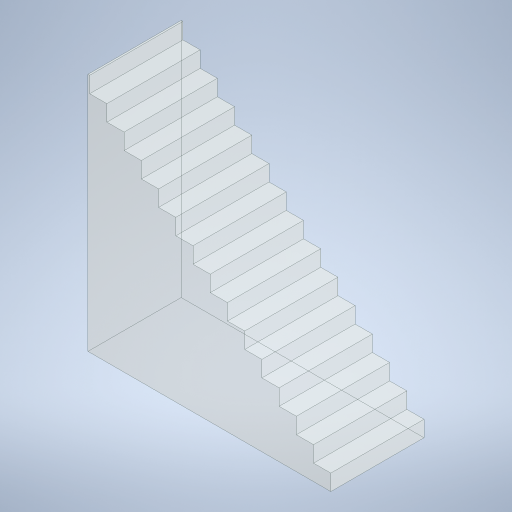
# Autodesk Inventor part: Stairs_Between_Finished_Basement_And_First_Floor
Saved by Autodesk Inventor 2024 (Build 280153000, 153)
## iProperties
Created: 2023-05-16
Part Number: Stairs_Between_Finished_Basement_And_First_Floor
Material: Steel
Document SubType Name: Modeling
Designer: Tom
Density: 7.85 g/cm^3
Appearance: Clear
Mass: 2.17052e+07 g
Surface Area: 147038 cm^2
Volume: 2.765e+06 cm^3
Author: Tom
Autodesk Inventor part; units mm, degrees
ref_plane "YZ Plane" through (0, 0, 0) normal (1, 0, 0) x (0, 1, 0)
ref_plane "XZ Plane" through (0, 0, 0) normal (0, 1, 0) x (-1, 0, 0)
ref_plane "XY Plane" through (0, 0, 0) normal (0, 0, 1) x (1, 0, 0)
sketch "Sketch1" plane through (0, 0, 0) normal (0, 0, 1) x (1, 0, 0)
  line L0 (-190.0464, 176.53) -> (-190.0464, 353.06)
  line L1 (-190.0464, 353.06) -> (-380.0929, 353.06)
  line L2 (-380.0929, 353.06) -> (-380.0929, 529.59)
  line L3 (-380.0929, 529.59) -> (-570.1393, 529.59)
  line L4 (-570.1393, 529.59) -> (-570.1393, 706.12)
  line L5 (-570.1393, 706.12) -> (-760.1857, 706.12)
  line L6 (-760.1857, 706.12) -> (-760.1857, 882.65)
  line L7 (-760.1857, 882.65) -> (-950.2321, 882.65)
  line L8 (-950.2321, 882.65) -> (-950.2321, 1059.18)
  line L9 (-950.2321, 1059.18) -> (-1140.2786, 1059.18)
  line L10 (-1140.2786, 1059.18) -> (-1140.2786, 1235.71)
  line L11 (-1140.2786, 1235.71) -> (-1330.325, 1235.71)
  line L12 (-1330.325, 1235.71) -> (-1330.325, 1412.24)
  line L13 (-1330.325, 1412.24) -> (-1520.3714, 1412.24)
  line L14 (-1520.3714, 1412.24) -> (-1520.3714, 1588.77)
  line L15 (-1520.3714, 1588.77) -> (-1710.4179, 1588.77)
  line L16 (-1710.4179, 1588.77) -> (-1710.4179, 1765.3)
  line L17 (-1710.4179, 1765.3) -> (-1900.4643, 1765.3)
  line L18 (-1900.4643, 1765.3) -> (-1900.4643, 1941.83)
  line L19 (-1900.4643, 1941.83) -> (-2090.5107, 1941.83)
  line L20 (-2090.5107, 1941.83) -> (-2090.5107, 2118.36)
  line L21 (-2090.5107, 2118.36) -> (-2280.5571, 2118.36)
  line L22 (-2280.5571, 2118.36) -> (-2280.5571, 2294.89)
  line L23 (-2280.5571, 2294.89) -> (-2470.6036, 2294.89)
  line L24 (-190.0464, 176.53) -> (0, 176.53)
  line L25 (0, 176.53) -> (0, 0)
  line L26 (0, 0) -> (-2679.7, 0)
  line L27 (-2470.6036, 2294.89) -> (-2470.6036, 2471.42)
  line L28 (-2470.6036, 2471.42) -> (-2660.65, 2471.42)
  line L29 (-2660.65, 2471.42) -> (-2660.65, 2647.95)
  line L30 (-2660.65, 2647.95) -> (-2679.7, 2647.95)
  line L31 (-2679.7, 2647.95) -> (-2679.7, 0)
  point P0 (-2762.8302, 625.5305)
  dimension "d21" = 2647.95
  dimension "d22" = 2679.7
  dimension "d23" = 19.05
  constraints: 64 end point, 27 parallel, 26 perpendicular, 3 horizontal, 3 vertical, 1 coincident
  measures "d21" distance of L30.end L26.end
  measures "d22" distance of L25.end L26.end
  measures "d23" distance of L29.end L30.end
extrude "Extrusion1" add sketch "Sketch1" along normal blind 1028.7
body "Solid1"
